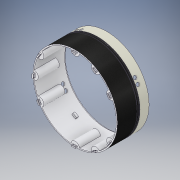
# Autodesk Inventor part: Than_new
Saved by Autodesk Inventor 2019 (Build 230136000, 136)
## iProperties
Created: 2021-01-14
Part Number: Than_new
Material: Polystyrene
Document SubType Name: Modeling
Designer: Admin
Density: 1.021 g/cm^3
Appearance: Weld - Aluminum
Author: Admin
Autodesk Inventor part; units mm, degrees
sketch "Sketch1" plane through (0, 0, 0) normal (0, 0, 1) x (1, 0, 0)
  circle A0 centre (0, 0) radius 200
  circle A1 centre (0, 0) radius 195
  dimension "d0" = 400
  dimension "d1" = 390
  constraints: 2 centre point, 2 coincident
  measures "d0" diameter of A0
  measures "d1" diameter of A1
extrude "Extrusion1" add sketch "Sketch1" along normal blind 150
ref_plane "Work Plane1" through (0, 0, 50) normal (0, 0, 1) x (1, 0, 0)
sketch "Sketch2" plane through (0, 0, 50) normal (0, 0, 1) x (1, 0, 0)
  circle A0 centre (0, 0) radius 200
  circle A1 centre (0, 0) radius 197.5
  dimension "d5" = 395
  constraints: 2 centre point, 2 coincident
  measures "d5" diameter of A1
extrude "Extrusion2" cut sketch "Sketch2" along normal mid plane 10
fillet "Fillet1" radius 2 4 edges at (-200, 0, 45) (-197.5, 0, 45) (-200, 0, 55) (-197.5, 0, 55)
sketch "Sketch3" plane through (0, 0, 150) normal (0, 0, 1) x (1, 0, 0)
  arc A0 (173.6513, 88.7144) -> (163.6545, 106.0292) centre (0, 0) ccw
  arc A1 (106.0292, 163.6545) -> (88.7144, 173.6513) centre (0, 0) ccw
  arc A2 (9.9967, 194.7436) -> (-9.9967, 194.7436) centre (0, 0) ccw
  arc A3 (-163.6545, 106.0292) -> (-173.6513, 88.7144) centre (0, 0) ccw
  arc A4 (-194.7436, 9.9967) -> (-194.7436, -9.9967) centre (0, 0) ccw
  arc A5 (-173.6513, -88.7144) -> (-163.6545, -106.0292) centre (0, 0) ccw
  arc A6 (-9.9967, -194.7436) -> (9.9967, -194.7436) centre (0, 0) ccw
  arc A7 (88.7144, -173.6513) -> (106.0292, -163.6545) centre (0, 0) ccw
  arc A8 (163.6545, -106.0292) -> (173.6513, -88.7144) centre (0, 0) ccw
  arc A9 (177.9736, -79.6895) -> (157.9999, -114.2849) centre (168.875, -97.5) ccw
  arc A10 (114.2849, -157.9999) -> (79.6895, -177.9736) centre (97.5, -168.875) ccw
  arc A11 (19.9737, -193.9744) -> (-19.9737, -193.9744) centre (0, -195) ccw
  arc A12 (157.9999, 114.2849) -> (177.9736, 79.6895) centre (168.875, 97.5) ccw
  arc A13 (79.6895, 177.9736) -> (114.2849, 157.9999) centre (97.5, 168.875) ccw
  arc A14 (-19.9852, 193.9732) -> (19.9852, 193.9732) centre (0, 194.7436) ccw
  arc A15 (-193.9744, -19.9737) -> (-193.9744, 19.9737) centre (-195, 0) ccw
  arc A16 (-177.9736, 79.6895) -> (-157.9999, 114.2849) centre (-168.875, 97.5) ccw
  arc A17 (-157.9999, -114.2849) -> (-177.9736, -79.6895) centre (-168.875, -97.5) ccw
  arc A18 (79.6895, -177.9736) -> (114.2849, -157.9999) centre (0, 0) ccw
  arc A19 (157.9999, -114.2849) -> (177.9736, -79.6895) centre (0, 0) ccw
  arc A20 (177.9736, 79.6895) -> (157.9999, 114.2849) centre (0, 0) ccw
  arc A21 (114.2849, 157.9999) -> (79.6895, 177.9736) centre (0, 0) ccw
  arc A22 (19.9852, 193.9732) -> (-19.9852, 193.9732) centre (0, 0) ccw
  arc A23 (-157.9999, 114.2849) -> (-177.9736, 79.6895) centre (0, 0) ccw
  arc A24 (-193.9744, 19.9737) -> (-193.9744, -19.9737) centre (0, 0) ccw
  arc A25 (-177.9736, -79.6895) -> (-157.9999, -114.2849) centre (0, 0) ccw
  arc A26 (-19.9737, -193.9744) -> (19.9737, -193.9744) centre (0, 0) ccw
  dimension "d22" = 40
  dimension "d23" = 40
  dimension "d24" = 40
  dimension "d25" = 40
  dimension "d26" = 40
  dimension "d27" = 40
  dimension "d28" = 40
  dimension "d29" = 40
  dimension "d30" = 40
  constraints: 54 point on circle, 27 centre point, 2 coincident
  measures "d22" diameter of A9
  measures "d23" diameter of A10
  measures "d24" diameter of A11
  measures "d25" diameter of A12
  measures "d26" diameter of A13
  measures "d27" diameter of A14
  measures "d28" diameter of A15
  measures "d29" diameter of A16
  measures "d30" diameter of A17
extrude "Extrusion3" add sketch "Sketch3" against normal blind 100
sketch "Sketch4" plane through (0, 0, 50) normal (0, 0, 1) x (1, 0, 0)
  line L0 (185, 0) -> (185, 10)
  line L1 (185, 10) -> (195, 10)
  line L2 (195, 10) -> (195, 0)
  line L3 (185, 0) -> (185, -10)
  line L4 (185, -10) -> (195, -10)
  line L5 (195, -10) -> (195, 0)
  line L6 (-92.5, 160.2147) -> (-101.1603, 155.2147)
  line L7 (-101.1603, 155.2147) -> (-106.1603, 163.875)
  line L8 (-106.1603, 163.875) -> (-97.5, 168.875)
  line L9 (-92.5, 160.2147) -> (-83.8397, 165.2147)
  line L10 (-83.8397, 165.2147) -> (-88.8397, 173.875)
  line L11 (-88.8397, 173.875) -> (-97.5, 168.875)
  line L12 (-92.5, -160.2147) -> (-83.8397, -165.2147)
  line L13 (-83.8397, -165.2147) -> (-88.8397, -173.875)
  line L14 (-88.8397, -173.875) -> (-97.5, -168.875)
  line L15 (-92.5, -160.2147) -> (-101.1603, -155.2147)
  line L16 (-101.1603, -155.2147) -> (-106.1603, -163.875)
  line L17 (-106.1603, -163.875) -> (-97.5, -168.875)
  line L18 (-101.1603, 155.2147) -> (-83.8397, 165.2147)
  line L19 (-88.8397, 173.875) -> (-106.1603, 163.875)
  circle A0 centre (-95, -164.5448) radius 1.5
  circle A1 centre (190, 0) radius 1.5
  point P0 (0, 0)
  point P1 (173.6513, 88.7144)
  point P2 (173.6513, -88.7144)
  point P3 (0, 0)
  dimension "d18" = 360
  dimension "d38" = 3
  constraints: 40 end point, 2 centre point, 1 coincident, 1 collinear, 1 parallel, 37 other
  measures "d38" diameter of A0
extrude "Extrusion4" add sketch "Sketch4" along normal blind 10 contours L0 L1 L2 L5 L4 L3 | L12 L13 L14 L17 L16 L15 | A0 | A1
extrude "Extrusion6" cut sketch "Sketch4" along normal blind 5 contours A0
extrude "Extrusion7" cut sketch "Sketch4" along normal blind 5 contours A1
sketch "Sketch6" plane through (0, 0, 150) normal (0, 0, 1) x (1, 0, 0)
  line L0 (0, -195) -> (-10, -195)
  line L1 (-10, -195) -> (-10, -190)
  line L2 (-10, -190) -> (0, -190)
  line L3 (0, -195) -> (10, -195)
  line L4 (10, -195) -> (10, -190)
  line L5 (10, -190) -> (0, -190)
  line L6 (106.1603, -163.875) -> (103.6603, -159.5448)
  line L7 (97.5, -168.875) -> (106.1603, -163.875)
  line L8 (97.5, -168.875) -> (88.8397, -173.875)
  line L9 (88.8397, -173.875) -> (86.3397, -169.5448)
  line L10 (86.3397, -169.5448) -> (95, -164.5448)
  line L11 (103.6603, -159.5448) -> (95, -164.5448)
  line L12 (173.875, -88.8397) -> (169.5448, -86.3397)
  line L13 (168.875, -97.5) -> (173.875, -88.8397)
  line L14 (168.875, -97.5) -> (163.875, -106.1603)
  line L15 (163.875, -106.1603) -> (159.5448, -103.6603)
  line L16 (159.5448, -103.6603) -> (164.5448, -95)
  line L17 (169.5448, -86.3397) -> (164.5448, -95)
  line L18 (195, 10) -> (190, 10)
  line L19 (195, 0) -> (195, 10)
  line L20 (195, 0) -> (195, -10)
  line L21 (195, -10) -> (190, -10)
  line L22 (190, -10) -> (190, 0)
  line L23 (190, 10) -> (190, 0)
  line L24 (163.875, 106.1603) -> (159.5448, 103.6603)
  line L25 (168.875, 97.5) -> (163.875, 106.1603)
  line L26 (168.875, 97.5) -> (173.875, 88.8397)
  line L27 (173.875, 88.8397) -> (169.5448, 86.3397)
  line L28 (169.5448, 86.3397) -> (164.5448, 95)
  line L29 (159.5448, 103.6603) -> (164.5448, 95)
  line L30 (88.8397, 173.875) -> (86.3397, 169.5448)
  line L31 (97.5, 168.875) -> (88.8397, 173.875)
  line L32 (97.5, 168.875) -> (106.1603, 163.875)
  line L33 (106.1603, 163.875) -> (103.6603, 159.5448)
  line L34 (103.6603, 159.5448) -> (95, 164.5448)
  line L35 (86.3397, 169.5448) -> (95, 164.5448)
  line L36 (-10, 195) -> (-10, 190)
  line L37 (0, 195) -> (-10, 195)
  line L38 (0, 195) -> (10, 195)
  line L39 (10, 195) -> (10, 190)
  line L40 (10, 190) -> (0, 190)
  line L41 (-10, 190) -> (0, 190)
  line L42 (-106.1603, 163.875) -> (-103.6603, 159.5448)
  line L43 (-97.5, 168.875) -> (-106.1603, 163.875)
  line L44 (-97.5, 168.875) -> (-88.8397, 173.875)
  line L45 (-88.8397, 173.875) -> (-86.3397, 169.5448)
  line L46 (-86.3397, 169.5448) -> (-95, 164.5448)
  line L47 (-103.6603, 159.5448) -> (-95, 164.5448)
  line L48 (-173.875, 88.8397) -> (-169.5448, 86.3397)
  line L49 (-168.875, 97.5) -> (-173.875, 88.8397)
  line L50 (-168.875, 97.5) -> (-163.875, 106.1603)
  line L51 (-163.875, 106.1603) -> (-159.5448, 103.6603)
  line L52 (-159.5448, 103.6603) -> (-164.5448, 95)
  line L53 (-169.5448, 86.3397) -> (-164.5448, 95)
  line L54 (-195, -10) -> (-190, -10)
  line L55 (-195, 0) -> (-195, -10)
  line L56 (-195, 0) -> (-195, 10)
  line L57 (-195, 10) -> (-190, 10)
  line L58 (-190, 10) -> (-190, 0)
  line L59 (-190, -10) -> (-190, 0)
  line L60 (-163.875, -106.1603) -> (-159.5448, -103.6603)
  line L61 (-168.875, -97.5) -> (-163.875, -106.1603)
  line L62 (-168.875, -97.5) -> (-173.875, -88.8397)
  line L63 (-173.875, -88.8397) -> (-169.5448, -86.3397)
  line L64 (-169.5448, -86.3397) -> (-164.5448, -95)
  line L65 (-159.5448, -103.6603) -> (-164.5448, -95)
  line L66 (-88.8397, -173.875) -> (-86.3397, -169.5448)
  line L67 (-97.5, -168.875) -> (-88.8397, -173.875)
  line L68 (-97.5, -168.875) -> (-106.1603, -163.875)
  line L69 (-106.1603, -163.875) -> (-103.6603, -159.5448)
  line L70 (-103.6603, -159.5448) -> (-95, -164.5448)
  line L71 (-86.3397, -169.5448) -> (-95, -164.5448)
  line L72 (10, -195) -> (-10, -195)
  line L73 (-10, -195) -> (-10, -190)
  line L74 (-10, -190) -> (10, -190)
  line L75 (10, -190) -> (10, -195)
  line L76 (10, 195) -> (-10, 195)
  line L77 (-10, 195) -> (-10, 190)
  line L78 (-10, 190) -> (10, 190)
  line L79 (10, 190) -> (10, 195)
  line L80 (-168.875, -97.5) -> (-163.875, -106.1603)
  line L81 (-163.875, -106.1603) -> (-159.5448, -103.6603)
  line L82 (-159.5448, -103.6603) -> (-169.5448, -86.3397)
  line L83 (-169.5448, -86.3397) -> (-173.875, -88.8397)
  line L84 (-173.875, -88.8397) -> (-163.875, -106.1603)
  line L85 (-190, -10) -> (-195, -10)
  line L86 (-195, -10) -> (-195, 10)
  line L87 (-195, 10) -> (-190, 10)
  line L88 (-190, 10) -> (-190, -10)
  line L89 (-159.5448, 103.6603) -> (-169.5448, 86.3397)
  line L90 (-159.5448, 103.6603) -> (-169.5448, 86.3397)
  line L91 (10, 195) -> (10, 190)
  line L92 (10, 190) -> (-10, 190)
  line L93 (-10, 190) -> (-10, 195)
  line L94 (106.1603, 163.875) -> (103.6603, 159.5448)
  line L95 (103.6603, 159.5448) -> (86.3397, 169.5448)
  line L96 (106.1603, 163.875) -> (88.8397, 173.875)
  line L97 (163.875, 106.1603) -> (159.5448, 103.6603)
  line L98 (173.875, -88.8397) -> (169.5448, -86.3397)
  line L99 (106.1603, -163.875) -> (103.6603, -159.5448)
  line L100 (103.6603, -159.5448) -> (86.3397, -169.5448)
  line L101 (88.8397, -173.875) -> (106.1603, -163.875)
  line L102 (-163.875, 106.1603) -> (-159.5448, 103.6603)
  line L103 (-159.5448, 103.6603) -> (-169.5448, 86.3397)
  line L104 (-169.5448, 86.3397) -> (-173.875, 88.8397)
  line L105 (88.8397, 173.875) -> (86.3397, 169.5448)
  line L106 (163.875, -106.1603) -> (159.5448, -103.6603)
  line L107 (159.5448, -103.6603) -> (169.5448, -86.3397)
  line L108 (169.5448, -86.3397) -> (173.875, -88.8397)
  line L109 (-163.875, 106.1603) -> (-173.875, 88.8397)
  line L110 (-163.875, 106.1603) -> (-173.875, 88.8397)
  line L111 (173.875, 88.8397) -> (169.5448, 86.3397)
  line L112 (169.5448, 86.3397) -> (159.5448, 103.6603)
  line L113 (163.875, 106.1603) -> (173.875, 88.8397)
  line L114 (163.875, -106.1603) -> (173.875, -88.8397)
  line L115 (173.875, -88.8397) -> (169.5448, -86.3397)
  line L116 (86.3397, -169.5448) -> (88.8397, -173.875)
  point P0 (0, 0)
  point P1 (0, 0)
  dimension "d44" = 10
  dimension "d45" = 5
  dimension "d48" = 360
  constraints: 234 end point, 16 collinear, 11 perpendicular, 7 parallel, 5 point on line, 3 horizontal, 1 vertical, 145 other
  measures "d44" distance of L1.end L2.end
  measures "d45" distance of L0.end L1.end
extrude "Extrusion8" add sketch "Sketch6" along normal blind 10 contours L0 L1 L2 L5 L4 L3 | L7 L8 L9 L10 L11 L6 | L13 L14 L15 L16 L17 L12 | L25 L26 L27 L28 L29 L24 | L31 L32 L33 L34 L35 L30 | L37 L38 L39 L40 L41 L36 | L49 L50 L51 L52 L53 L48 | L55 L56 L57 L58 L59 L54 | L61 L62 L63 L64 L65 L60
sketch "Sketch7" plane through (-163.875, -106.1603, 150) normal (-0.866, -0.5, 0) x (0, 0, 1)
  line L0 (0, 20) -> (0, 0) projected
  line L1 (10, 0) -> (10, 20) projected
  line L2 (7.5, 2.5) -> (2.5, 2.5)
  line L3 (2.5, 2.5) -> (2.5, 17.5)
  line L4 (2.5, 17.5) -> (7.5, 17.5)
  line L5 (7.5, 17.5) -> (7.5, 2.5)
  point P0 (-150, 10)
  dimension "d52" = 5
  dimension "d53" = 15
  constraints: 8 end point, 2 parallel, 1 horizontal, 1 perpendicular
  measures "d52" distance of L3.end L4.end
  measures "d53" distance of L2.end L3.end
extrude "Extrusion9" cut sketch "Sketch7" against normal blind 1000
sketch "Sketch8" plane through (-195, -10, 150) normal (-1, 0, 0) x (0, 0, 1)
  line L0 (0, 89.6895) -> (0, -69.6895) projected
  line L1 (7.5, 2.5) -> (2.5, 2.5)
  line L2 (2.5, 2.5) -> (2.5, 17.5)
  line L3 (2.5, 17.5) -> (7.5, 17.5)
  line L4 (7.5, 17.5) -> (7.5, 2.5)
  line L5 (7.5, 2.5) -> (2.5, 17.5) construction
  line L6 (2.5, 2.5) -> (7.5, 17.5) construction
  point P0 (-150, 10)
  point P1 (0, 0)
  point P2 (5, 10)
  dimension "d56" = 5
  dimension "d57" = 15
  constraints: 12 end point, 2 midpoint, 2 parallel, 1 horizontal, 1 perpendicular
  measures "d56" distance of L2.end L3.end
  measures "d57" distance of L1.end L2.end
extrude "Extrusion10" cut sketch "Sketch8" against normal blind 1000
sketch "Sketch9" plane through (-173.875, 88.8397, 150) normal (-0.866, 0.5, 0) x (0, 0, 1)
  line L0 (0, 0) -> (10, 0) projected
  line L1 (2.5, 2.5) -> (7.5, 2.5)
  line L2 (7.5, 2.5) -> (7.5, 17.5)
  line L3 (7.5, 17.5) -> (2.5, 17.5)
  line L4 (2.5, 17.5) -> (2.5, 2.5)
  line L5 (2.5, 2.5) -> (7.5, 17.5) construction
  line L6 (7.5, 2.5) -> (2.5, 17.5) construction
  point P0 (-150, 10)
  point P1 (10, 20)
  point P2 (0, 20)
  point P3 (5, 10)
  dimension "d60" = 5
  constraints: 12 end point, 2 midpoint, 2 parallel, 1 horizontal, 1 perpendicular
  measures "d60" distance of L3.end L2.end
extrude "Extrusion11" cut sketch "Sketch9" against normal blind 1000
sketch "Sketch10" plane through (-10, 195, 150) normal (0, 1, 0) x (1, 0, 0)
  line L0 (2.5, -2.5) -> (17.5, -2.5)
  line L1 (17.5, -2.5) -> (17.5, -7.5)
  line L2 (17.5, -7.5) -> (2.5, -7.5)
  line L3 (2.5, -7.5) -> (2.5, -2.5)
  line L4 (2.5, -2.5) -> (17.5, -7.5) construction
  line L5 (17.5, -2.5) -> (2.5, -7.5) construction
  point P0 (10, 150)
  point P1 (20, 0)
  point P2 (20, -10)
  point P3 (10, -5)
  dimension "d65" = 5
  constraints: 12 end point, 2 midpoint, 2 parallel, 1 horizontal, 1 perpendicular
  measures "d65" distance of L0.end L1.end
extrude "Extrusion12" cut sketch "Sketch10" against normal blind 1000
sketch "Sketch11" plane through (88.8397, 173.875, 160) normal (0.5, 0.866, 0) x (0.866, -0.5, 0)
  line L0 (2.5, 7.5) -> (17.5, 7.5)
  line L1 (17.5, 7.5) -> (17.5, 2.5)
  line L2 (17.5, 2.5) -> (2.5, 2.5)
  line L3 (2.5, 2.5) -> (2.5, 7.5)
  line L4 (2.5, 7.5) -> (17.5, 2.5) construction
  line L5 (17.5, 7.5) -> (2.5, 2.5) construction
  point P0 (10, 160)
  point P1 (10, 5)
  dimension "d68" = 15
  dimension "d69" = 5
  constraints: 12 end point, 2 midpoint, 2 parallel, 1 horizontal, 1 perpendicular
  measures "d68" distance of L1.end L2.end
  measures "d69" distance of L0.end L1.end
extrude "Extrusion13" cut sketch "Sketch11" against normal blind 1000
sketch "Sketch12" plane through (106.1603, -163.875, 150) normal (0.5, -0.866, 0) x (0.866, 0.5, 0)
  line L0 (190, 0) -> (-210, 0) projected
  line L1 (-2.5, 2.5) -> (-17.5, 2.5)
  line L2 (-17.5, 2.5) -> (-17.5, 7.5)
  line L3 (-17.5, 7.5) -> (-2.5, 7.5)
  line L4 (-2.5, 7.5) -> (-2.5, 2.5)
  line L5 (-2.5, 2.5) -> (-17.5, 7.5) construction
  line L6 (-17.5, 2.5) -> (-2.5, 7.5) construction
  point P0 (-10, -150)
  point P1 (-10, 5)
  dimension "d72" = 15
  dimension "d73" = 5
  constraints: 12 end point, 2 midpoint, 2 parallel, 1 horizontal, 1 perpendicular
  measures "d72" distance of L2.end L3.end
  measures "d73" distance of L1.end L2.end
extrude "Extrusion14" cut sketch "Sketch12" against normal blind 1000
sketch "Sketch13" plane through (0, 0, 0) normal (0, 0, -1) x (-1, 0, 0)
  circle A0 centre (0, 0) radius 197.5
  circle A1 centre (0, 0) radius 195
  dimension "d76" = 395
  dimension "d77" = 390
  constraints: 2 centre point, 2 coincident
  measures "d76" diameter of A0
  measures "d77" diameter of A1
extrude "Extrusion15" cut sketch "Sketch13" against normal blind 5
ref_plane "Work Plane2" through (-100, 173.2051, 0) normal (0.5, -0.866, 0) x (0.866, 0.5, 0)
sketch "Sketch14" plane through (-100, 173.2051, 0) normal (0.5, -0.866, 0) x (0.866, 0.5, 0)
  circle A0 centre (-12.75, 33) radius 8
  circle A1 centre (12.75, 33) radius 8
  point P0 (0, 0)
  dimension "d82" = 16
  constraints: 2 centre point
  measures "d82" diameter of A0
extrude "Extrusion16" cut sketch "Sketch14" along normal blind 1000
ref_plane "Work Plane5" through (173.2051, 100, 0) normal (-0.866, -0.5, 0) x (0.5, -0.866, 0)
sketch "Sketch15" plane through (173.2051, 100, 0) normal (-0.866, -0.5, 0) x (0.5, -0.866, 0)
  circle A0 centre (12.75, 33) radius 8
  circle A1 centre (-12.75, 33) radius 8
  point P0 (0, 0)
  dimension "d87" = 16
  constraints: 2 centre point
  measures "d87" diameter of A0
extrude "Extrusion17" cut sketch "Sketch15" along normal blind 1000
body "Solid1"
